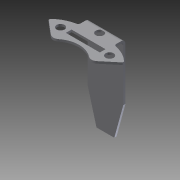
# Autodesk Inventor part: ASAP_Handle_Fixture_New2
Saved by Autodesk Inventor 2011 SP2 (Build 150309200, 309)
## iProperties
Created: 2012-02-26
Part Number: ASAP_Handle_Fixture_New2
Material: Default
Document SubType Name: Sheet Metal
Designer: sungwook
Density: 1 g/cm^3
Sheet Metal Rule: Default_mm
Author: sungwook
Autodesk Inventor part; units mm, degrees
ref_plane "YZ Plane" through (0, 0, 0) normal (1, 0, 0) x (0, 1, 0)
ref_plane "XZ Plane" through (0, 0, 0) normal (0, 1, 0) x (-1, 0, 0)
ref_plane "XY Plane" through (0, 0, 0) normal (0, 0, 1) x (1, 0, 0)
sketch "Sketch1" plane through (0, 0, 0) normal (0, 0, 1) x (1, 0, 0)
  circle A0 centre (0, 0) radius 0.889
  circle A1 centre (5.5, -3.27) radius 0.889
  circle A2 centre (-5.5, -3.27) radius 0.889
  line L0 (3.81, -2.5) -> (3.81, -3.77)
  line L1 (3.81, -3.77) -> (-3.81, -3.77)
  line L2 (-3.81, -3.77) -> (-3.81, -2.5)
  line L3 (-3.81, -2.5) -> (3.81, -2.5)
  line L4 (4, 1.7859) -> (4, -0.2965)
  line L5 (4, 1.7859) -> (-4, 1.7859)
  line L6 (-4, -0.2965) -> (-4, 1.7859)
  arc A3 (-4.4226, -0.8069) -> (-4, -0.2965) centre (-4.5195, -0.2965) ccw
  arc A4 (-4.4226, -0.8069) -> (-8.125, -2.6612) centre (-2.9898, -8.291) ccw
  arc A5 (-8.125, -2.6612) -> (-8.165, -3.2687) centre (-7.9224, -2.9796) ccw
  line L7 (-8.165, -3.2687) -> (-5.1371, -5.8094)
  arc A6 (-5.1371, -5.8094) -> (-3.4399, -5.8285) centre (-4.2769, -4.7842) ccw
  arc A7 (3.4399, -5.8285) -> (-3.4399, -5.8285) centre (0, -10.12) ccw
  arc A8 (3.4399, -5.8285) -> (5.1371, -5.8094) centre (4.2769, -4.7842) ccw
  line L8 (5.1371, -5.8094) -> (8.165, -3.2687)
  arc A9 (8.165, -3.2687) -> (8.125, -2.6612) centre (7.9224, -2.9796) ccw
  arc A10 (8.125, -2.6612) -> (4.4226, -0.8069) centre (2.9898, -8.291) ccw
  arc A11 (4, -0.2965) -> (4.4226, -0.8069) centre (4.5195, -0.2965) ccw
  line L9 (-11.6467, 0) -> (11.6467, 0)
  point P0 (0, 3.6369)
  dimension "d3" = 1.7859
  measures "d3" distance between parallel lines of L9 L5
extrude "Plate1" add sketch "Sketch1" along normal blind 0.5 contours L9 L4 A11 A10 A9 L8 A8 A7 A6 L7 A5 A4 A3 L6 A0 | A0 L9 L6 L5 L4
sketch "Sketch2" plane through (-4, 1.2859, 0.5) normal (0, 1, 0) x (-1, 0, 0)
  line L0 (-8, 0) -> (0, 0)
  line L1 (0, 0) -> (0, 20)
  line L2 (0, 20) -> (-8, 20)
  line L3 (-8, 20) -> (-8, 0)
  constraints: 4 end point, 4 other
edge flange "Flange1" height 20 angle -90 thickness 0.5 bend radius 0.5 thickness toward (0, 1, 0) relief straight relief width 0.5 relief depth 0.25 edges at (0, 1.7859, 0.5) wall of the first edge with corners at (4, 1.2859, 0.5) (-4, 1.2859, 0.5) (-4, 1.2859, -19.5) (4, 1.2859, -19.5)
bend "Bend1"
corner "Corner1"
sketch "Sketch3" plane through (-4, 1.7859, -19.5) normal (0, 1, 0) x (1, 0, 0)
  line L0 (0, 0) -> (8, 0)
  line L1 (8, 0) -> (8, -20)
  line L2 (8, -20) -> (0, -20)
  line L3 (0, -20) -> (0, 0)
  line L4 (2, 0) -> (0, -7.32)
  line L5 (6, 0) -> (8, -7.32)
  point P0 (4, -19.5)
  point P1 (4, -10)
  point P2 (4, 0)
  point P3 (0, -10)
  dimension "d14" = 8
  dimension "d15" = 20
  dimension "d16" = 7.32
  dimension "d17" = 2
  dimension "d18" = 7.32
  dimension "d19" = 4
  constraints: 12 end point, 4 point on line, 2 midpoint, 2 parallel, 1 horizontal, 1 horizontal alignment, 1 perpendicular, 1 vertical alignment
  measures "d14" distance between parallel lines of L1 L3
  measures "d15" distance between parallel lines of L2 L0
  measures "d16" vertical distance of L4.end L4.start
  measures "d17" distance of point (4, 0) L4.start
  measures "d18" vertical distance of L5.end L5.start
  measures "d19" distance of L5.start L4.start
extrude "Cut1" cut sketch "Sketch3" against normal blind 0.5 contours L0 L4 L3 | L0 L1 L5
equation "\"d20\" = Thickness"
equation "\"d4\" = BendReliefWidth"
equation "\"d5\" = BendReliefDepth"
equation "\"d6\" = MinimumRemnant"
equation "\"d7\" = BendRadius"
equation "\"d10\" = BendRadius"
equation "\"d11\" = CornerReliefSize"
equation "\"d12\" = GapSize"
equation "\"d13\" = JacobiRadiusSize"
equation "\"BendRadius\" = Thickness"
equation "\"BendReliefWidth\" = Thickness"
equation "\"BendReliefDepth\" = 0.5 * Thickness"
equation "\"CornerReliefSize\" = 4 * Thickness"
equation "\"MinimumRemnant\" = 2 * Thickness"
equation "\"TransitionRadius\" = BendRadius"
equation "\"JacobiRadiusSize\" = BendRadius"
equation "\"GapSize\" = Thickness"
equation "\"d0\" = BendRadius"
equation "\"Thickness\" = 0.5"
body "Solid1"
